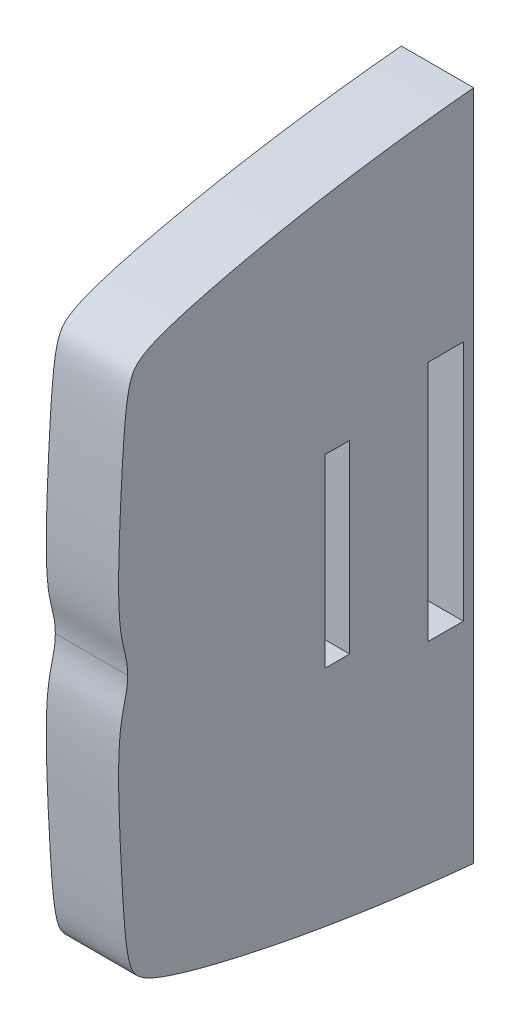
# Autodesk Inventor part: Interface_Left_Pannel
Saved by Autodesk Inventor 2016 (Build 200138000, 138)
## iProperties
Created: 2015-06-09
Part Number: Interface_Left_Pannel
Material: ABS Plastic
Document SubType Name: Modeling
Designer: Yann
Density: 1.06 g/cm^3
Appearance: Smooth - White
Author: Yann
Autodesk Inventor part; units mm, degrees
ref_plane "YZ Plane" through (0, 0, 0) normal (1, 0, 0) x (0, 1, 0)
ref_plane "XZ Plane" through (0, 0, 0) normal (0, 1, 0) x (-1, 0, 0)
ref_plane "XY Plane" through (0, 0, 0) normal (0, 0, 1) x (1, 0, 0)
sketch "Sketch1" plane through (0, 0, 0) normal (1, 0, 0) x (0, 1, 0)
  line L0 (-11.5, 1.2) -> (-11.5, 4.2) construction
  line L1 (11.5, 1.2) -> (11.5, 4.2) construction
  line L2 (0, 56.2307) -> (0, -9.9122) construction
  line L3 (-11.5, 2.7) -> (0, 2.7) construction
  line L4 (11.7, 1) -> (-11.7, 1)
  line L5 (-11.7, 1) -> (-11.7, 4.4)
  line L6 (-11.7, 4.4) -> (11.7, 4.4)
  line L7 (11.7, 4.4) -> (11.7, 1)
  line L8 (11.7, 1) -> (-11.7, 4.4) construction
  line L9 (-11.7, 1) -> (11.7, 4.4) construction
  spline S0 degree 3 poles (-32.5, 0) (-31.26, 12.9744) (-29.1717, 22.3157) (-27.1997, 29.671) (-26.6515, 30.9429) (-25.9975, 32.1759) (-25.73, 32.4921) (-25.3073, 32.8507) (-25.0652, 33.0052) (-24.1345, 33.3491) (-23.3821, 33.4996) (-19.5208, 33.9791) (-11.9188, 34.3204) (-6.4023, 34.3801) (-4.7631, 34.2962) (-2.0832, 33.8297) (-1.3517, 33.4863) (0, 33.4863) knots 0 0 0 0 3.910045 3.910045 6.649541 6.649541 9.041662 9.041662 10.846699 10.846699 13.376814 13.376814 20.536367 20.536367 25.926986 25.926986 31.518877 31.518877 31.518877 31.518877 projected
  spline S1 degree 3 poles (0, 33.4863) (0.9863, 33.4863) (1.6753, 33.669) (3.779, 34.1784) (5.346, 34.4656) (13.3886, 34.2388) (19.0102, 33.9988) (23.488, 33.5047) (24.4444, 33.2965) (25.3319, 32.8426) (25.5605, 32.6625) (26.073, 32.0547) (26.3494, 31.5594) (27.5158, 28.8658) (28.3939, 25.2853) (29.7852, 19.106) (31.4224, 11.2744) (32.5, 0) knots 0 0 0 0 0.295882 0.295882 0.869547 0.869547 1.170927 1.170927 1.327498 1.327498 1.401763 1.401763 1.502384 1.502384 1.834177 1.834177 2.289619 2.289619 2.289619 2.289619 projected
  line L10 (-32.5, 0) -> (32.5, 0)
  line L11 (-8.75, 12.2) -> (-8.75, 14.2) construction
  line L12 (8.75, 12.2) -> (8.75, 14.2) construction
  line L13 (-8.75, 13.2) -> (8.75, 13.2) construction
  line L14 (8.95, 12) -> (-8.95, 12)
  line L15 (-8.95, 12) -> (-8.95, 14.4)
  line L16 (-8.95, 14.4) -> (8.95, 14.4)
  line L17 (8.95, 14.4) -> (8.95, 12)
  line L18 (8.95, 12) -> (-8.95, 14.4) construction
  line L19 (-8.95, 12) -> (8.95, 14.4) construction
  point P0 (0, 0)
  point P1 (0, 13.2)
  dimension "d0" = 0.2
  dimension "d1" = 0.2
  dimension "d2" = 0.2
  dimension "d3" = 0.2
  constraints: 30 end point, 8 midpoint, 4 horizontal, 4 parallel, 3 perpendicular, 1 point on line
  measures "d0" distance between parallel lines of L5 L0
  measures "d1" distance from line of L0.end L6
  measures "d2" distance from line of L13.start L15
  measures "d3" distance from line of L11.end L16
extrude "Extrusion1" add sketch "Sketch1" against normal blind 7
equation "\"d2\" = d1"
equation "\"d3\" = d2"
equation "\"d4\" = Interface_Thickness"
equation "\"Heatsink_Thickness\" = 5"
equation "\"Heatsink_Width\" = 65"
equation "\"Cover_Thickness\" = 2"
equation "\"PowerPCB_Minus_Height\" = 1.2"
equation "\"PowerPCB_Width\" = 63"
equation "\"Interface_Thickness\" = 7"
equation "\"PowerPCB_Thickness\" = 3"
equation "\"PowerPCB_Plus_Height\" = 8"
equation "\"LogicPCB_Width\" = 55"
equation "\"LogicPCB_Thickness\" = 2"
equation "\"LogicPCB_Plus_Height\" = 8"
equation "\"HostPCB_Thickness\" = 1.2"
equation "\"HostPCB_Plus_Height\" = 8"
body "Solid1"
